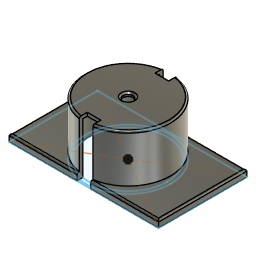
Magnet Holder v4 (Autodesk Fusion 360 design; units mm, degrees)
Autodesk Fusion 360 part; units mm, degrees
sketch "Sketch1" plane through (0, 0, 0) normal (0, 0, 1) x (1, 0, 0)
  circle A0 centre (0, 0) radius 11.5
  circle A1 centre (0, 0) radius 12.5
  line L0 (22, -13) -> (-22, -13)
  line L1 (-22, -13) -> (-22, 13)
  line L2 (-22, 13) -> (22, 13)
  line L3 (22, 13) -> (22, -13)
  line L4 (22, -13) -> (-22, 13) construction
  line L5 (-22, -13) -> (22, 13) construction
  constraint coincident A0.centre A1.centre
  constraint horizontal L0
  constraint perpendicular L0 L1
  constraint parallel L0 L2
  constraint parallel L1 L3
  constraint coincident L4 A0.centre
  constraint coincident L5 A0.centre
extrude "Extrude22" add sketch "Sketch1" along normal blind 2 contours A1 | L0 L1 L2 L3
sketch "Sketch16" plane through (0, 0, 2) normal (0, 0, 1) x (-1, 0, 0)
  circle A0 centre (0, 0) radius 11.5
  line L0 (-22, -13) -> (22, -13)
  line L1 (22, -13) -> (22, 13)
  line L2 (22, 13) -> (-22, 13)
  line L3 (-22, 13) -> (-22, -13)
  circle A1 centre (0, 0) radius 12.5
  constraint coincident A0.centre A1.centre
extrude "Extrude23" add sketch "Sketch16" along normal blind 13 contours A1
sketch "Sketch17" plane through (0, 0, 15) normal (0, 0, 1) x (-1, 0, 0)
  circle A0 centre (0, 0) radius 11.5
  circle A1 centre (0, 0) radius 12.5
  circle A2 centre (0, 0) radius 12.5
  constraint coincident A0.centre A1.centre
extrude "Extrude24" add sketch "Sketch17" along normal blind 1 contours A0 | A1 A2
hole "Hole3" at (0, 0, 16) direction (0, 0, -1) diameter 3 depth 6 tip angle 180 countersink diameter 4 countersink angle 90
sketch "Sketch18" plane through (0, 0, 16) normal (0, 0, 1) x (-1, 0, 0)
  circle A0 centre (0, 0) radius 2
  circle A1 centre (0, 0) radius 12.5
  line L0 (2, 10) -> (-2, 10)
  line L1 (-2, 10) -> (-2, 14)
  line L2 (-2, 14) -> (2, 14)
  line L3 (2, 14) -> (2, 10)
  line L4 (2, -10) -> (-2, -10)
  line L5 (-2, -10) -> (-2, -14)
  line L6 (-2, -14) -> (2, -14)
  line L7 (2, -14) -> (2, -10)
  constraint horizontal L0
  constraint vertical L1
  constraint horizontal L2
  constraint vertical L3
  constraint horizontal L4
  constraint vertical L5
  constraint horizontal L6
  constraint vertical L7
extrude "Extrude25" cut sketch "Sketch18" against normal blind 16 contours A1 L0 L1 L3 | A1 L1 L2 L3 | A1 L5 L6 L7 | A1 L4 L5 L7
fillet "Fillet3" radius 0.5 2 edges at (12.5, 0, 16) (-12.5, 0, 16)
fillet "Fillet4" radius 0.5 3 edges at (12, 13, 2) (22, 0, 2) (12, -13, 2)
fillet "Fillet5" radius 0.5 3 edges at (-12, -13, 2) (-22, 0, 2) (-12, 13, 2)
extrude "Extrude17" [rolled back] along distance 2 taper angle 0
extrude "Extrude18" [rolled back] along distance 15.24 taper angle 0
sketch "Sketch14" plane through (0, 0, 15.24) normal (0, 0, 1) x (-1, 0, 0)
  circle A0 centre (0, 0) radius 10
  circle A1 centre (0, 0) radius 11
  circle A2 centre (0, 0) radius 11
  constraint coincident A0.centre A1.centre
extrude "Extrude19" [rolled back] along distance 1 taper angle 0
hole "Hole2" [rolled back] hole depth 6 hole diameter 0.9 tip angle 180 csdiameter 2.5 csangle 90
sketch "Sketch15" plane through (0, 0, 16.24) normal (0, 0, 1) x (-1, 0, 0)
  circle A0 centre (0, 0) radius 1.25
  circle A1 centre (0, 0) radius 11
  line L0 (2, 9) -> (-2, 9)
  line L1 (-2, 9) -> (-2, 13)
  line L2 (-2, 13) -> (2, 13)
  line L3 (2, 13) -> (2, 9)
  line L4 (2, -9) -> (-2, -9)
  line L5 (-2, -9) -> (-2, -13)
  line L6 (-2, -13) -> (2, -13)
  line L7 (2, -13) -> (2, -9)
  constraint horizontal L0
  constraint vertical L1
  constraint horizontal L2
  constraint vertical L3
  constraint horizontal L4
  constraint vertical L5
  constraint horizontal L6
  constraint vertical L7
extrude "Extrude20" [rolled back] along distance -8 taper angle 0
fillet "Fillet1" [rolled back] radius 0.5
fillet "Fillet2" [rolled back] radius 0.5
extrude "Extrude21" [rolled back] along distance 2 taper angle 0
extrude "Extrude1" [rolled back] side1wall thickness 1 along distance 20 taper angle 0
sketch "Sketch2" plane through (0, 0, 0) normal (0, 0, 1) x (1, 0, 0)
  line L0 (-5, -10) -> (5, -10)
  line L1 (-5, -10) -> (-5, -8.6603)
  line L2 (5, -10) -> (5, -8.6603)
  arc A0 (5, -8.6603) -> (-5, -8.6603) centre (0, 0) ccw
  constraint horizontal L0
  constraint coincident A0.centre origin
  constraint perpendicular L0 L1
  constraint perpendicular L0 L2
extrude "Extrude2" [rolled back] along distance 2.5 taper angle 0
ref_plane "WorkPlane1" through (0, 0, 17.5) normal (0, 0, 1) x (1, 0, 0)
sketch "Sketch3" plane through (0, 0, 17.5) normal (0, 0, 1) x (1, 0, 0)
sketch "Sketch4" plane through (0, 0, 2.5) normal (0, 0, 1) x (-1, 0, 0)
  line L0 (5, 10) -> (-5, 10)
  line L1 (-5, 10) -> (-5, 8.6603)
  arc A0 (-5, 8.6603) -> (5, 8.6603) centre (0, 0) ccw
  line L2 (5, 8.6603) -> (5, 10)
  line L3 (-14, 9) -> (-6.3275, 9)
  line L4 (-14, 9) -> (-14, 5.5247)
  spline S0 degree 5 poles (-14, 5.5247) (-13.9496, 5.4874) (-13.8498, 5.4119) (-13.7027, 5.2958) (-13.512, 5.1353) (-13.283, 4.9251) (-13.0636, 4.7056) (-12.8545, 4.4775) (-12.6567, 4.242) (-12.4712, 4.0012) (-12.2993, 3.7572) (-12.1415, 3.5119) (-11.9978, 3.2656) (-11.8668, 3.0169) (-11.7458, 2.762) (-11.6318, 2.4964) (-11.5225, 2.2153) (-11.4171, 1.9151) (-11.3178, 1.5946) (-11.2257, 1.2533) (-11.1416, 0.8912) (-11.0809, 0.5849) (-11.039, 0.346) (-11.0127, 0.1827) (-11, 0.1) knots 0 0 0 0 0 0 0.05 0.1 0.15 0.2 0.25 0.3 0.35 0.4 0.45 0.5 0.55 0.6 0.65 0.7 0.75 0.8 0.85 0.9 0.95 1 1 1 1 1 1
  line L5 (-11.6858, 2.681) -> (-11.25, 1.43)
  spline S1 degree 5 poles (-6.3275, 9) (-6.5288, 8.8498) (-6.9165, 8.549) (-7.4534, 8.096) (-8.0838, 7.4871) (-8.7489, 6.709) (-9.3131, 5.9024) (-9.7954, 5.0559) (-10.2069, 4.1611) (-10.5469, 3.2164) (-10.8062, 2.224) (-10.9382, 1.3948) (-10.9888, 0.7544) (-11, 0.3195) (-11, 0.1) knots 0 0 0 0 0 0 0.1 0.2 0.3 0.4 0.5 0.6 0.7 0.8 0.9 1 1 1 1 1 1
  line L6 (-5.255, 9.8) -> (-7.4, 8.2)
  line L7 (-11, 1.3) -> (-11, -1.1)
  point P0 (-12.87, 4.49)
  point P1 (-12.0347, 3.325)
  point P2 (-11.4679, 2.0555)
  point P3 (-9.8, 5)
  constraint horizontal L3
  constraint perpendicular L3 L4
  constraint midpoint P2 L5
  constraint midpoint L3.end L6
  constraint midpoint S0.end L7
extrude "Extrude3" [rolled back] along distance 2 taper angle 0
sketch "Sketch5" plane through (0, 0, 2.5) normal (0, 0, 1) x (-1, 0, 0)
  line L0 (5, 10) -> (-5, 10)
  line L1 (-5, 10) -> (-5, 8.6603)
  arc A0 (-5, 8.6603) -> (5, 8.6603) centre (0, 0) ccw
  line L2 (5, 8.6603) -> (5, 10)
  line L3 (14, 9) -> (6.3249, 9)
  line L4 (14, 9) -> (14, 5.52)
  spline S0 degree 5 poles (10.9999, 0.073) (11.0319, 0.2346) (11.0981, 0.5527) (11.204, 1.0147) (11.3588, 1.5997) (11.5765, 2.2762) (11.8213, 2.8939) (12.0963, 3.4498) (12.4047, 3.9441) (12.748, 4.3849) (13.1266, 4.7859) (13.458, 5.0862) (13.7227, 5.305) (13.9064, 5.4487) (14, 5.52) knots 0 0 0 0 0 0 0.1 0.2 0.3 0.4 0.5 0.6 0.7 0.8 0.9 1 1 1 1 1 1
  line L5 (13.4267, 5.0834) -> (14.5733, 5.9566)
  spline S1 degree 5 poles (10.9999, 0.073) (11.0009, 0.2091) (10.9984, 0.4805) (10.9814, 0.8857) (10.9323, 1.4218) (10.826, 2.0845) (10.6756, 2.7386) (10.4831, 3.3819) (10.2565, 4.0106) (9.9997, 4.6218) (9.7097, 5.2156) (9.3805, 5.7931) (9.0049, 6.356) (8.5777, 6.9061) (8.097, 7.445) (7.5628, 7.9736) (7.0933, 8.3887) (6.7181, 8.696) (6.4577, 8.899) (6.3249, 9) knots 0 0 0 0 0 0 0.066667 0.133333 0.2 0.266667 0.333333 0.4 0.466667 0.533333 0.6 0.666667 0.733333 0.8 0.866667 0.933333 1 1 1 1 1 1
  line L6 (10.848, 2.2166) -> (10.152, 4.3834)
  point P0 (12.2, 3.6)
  point P1 (10.5, 3.3)
  point P2 (9.1, 6.2)
  constraint parallel L0 L3
  constraint perpendicular L3 L4
  constraint midpoint L4.end L5
  constraint midpoint P1 L6
extrude "Extrude4" [rolled back] along distance 2 taper angle 0
ref_plane "WorkPlane2" through (0, 0, 17.5) normal (0, 0, 1) x (1, 0, 0)
sketch "Sketch6" plane through (0, 0, 17.5) normal (0, 0, 1) x (1, 0, 0)
sketch "Sketch7" plane through (0, 0, 0) normal (0, 0, 1) x (1, 0, 0)
hole "Hole1" [rolled back] hole depth 2 hole diameter 3 tip angle 118 cbdepth 1 cbdiameter 4
extrude "Extrude5" [rolled back] along distance 2.5 taper angle 0
extrude "Extrude6" [rolled back] along distance 2.5 taper angle 0
extrude "Extrude7" [rolled back] along distance -2 taper angle 0
extrude "Extrude8" [rolled back] along distance -2 taper angle 0
ref_plane "WorkPlane3" through (0, 0, 17.5) normal (0, 0, 1) x (1, 0, 0)
sketch "Sketch8" plane through (0, 0, 17.5) normal (0, 0, 1) x (1, 0, 0)
  line L0 (-14, -9) -> (-6.3251, -9)
  line L1 (-14, -9) -> (-14, -5.5188)
  spline S0 degree 5 poles (-14, -5.5188) (-13.9096, -5.4464) (-13.7383, -5.3073) (-13.5098, -5.1161) (-13.2493, -4.8848) (-12.9385, -4.5749) (-12.5913, -4.1764) (-12.1926, -3.6334) (-11.8154, -2.9315) (-11.4931, -2.1293) (-11.2439, -1.3171) (-11.1073, -0.7399) (-11.0401, -0.3851) (-11.0108, -0.1884) (-11, -0.1) knots 0 0 0 0 0 0 0.1 0.2 0.3 0.4 0.5 0.6 0.7 0.8 0.9 1 1 1 1 1 1
  line L2 (-14.61, -6.0076) -> (-13.39, -5.03)
  line L3 (-12.8121, -4.4826) -> (-11.9879, -3.3174)
  line L4 (-11.05, -0.51) -> (-10.95, 0.31)
  spline S1 degree 5 poles (-11, -0.1) (-10.9944, -0.2588) (-10.9791, -0.5743) (-10.9436, -1.0413) (-10.871, -1.6515) (-10.7372, -2.3925) (-10.5591, -3.1106) (-10.3363, -3.8043) (-10.0691, -4.4715) (-9.7604, -5.1102) (-9.4143, -5.7181) (-9.0362, -6.2933) (-8.6311, -6.8339) (-8.2039, -7.3388) (-7.758, -7.8078) (-7.296, -8.2418) (-6.9147, -8.5617) (-6.6223, -8.7866) (-6.4246, -8.93) (-6.3251, -9) knots 0 0 0 0 0 0 0.066667 0.133333 0.2 0.266667 0.333333 0.4 0.466667 0.533333 0.6 0.666667 0.733333 0.8 0.866667 0.933333 1 1 1 1 1 1
  point P0 (-12.4, -3.9)
  point P1 (-10.25, -4)
  point P2 (-8.5, -6.98)
  constraint horizontal L0
  constraint perpendicular L0 L1
  constraint midpoint L1.end L2
  constraint midpoint P0 L3
  constraint midpoint S0.end L4
extrude "Extrude9" [rolled back] along distance 2.5 taper angle 0
ref_plane "WorkPlane4" through (0, 0, 17.5) normal (0, 0, 1) x (1, 0, 0)
sketch "Sketch9" plane through (0, 0, 17.5) normal (0, 0, 1) x (1, 0, 0)
ref_plane "WorkPlane5" through (0, 0, 17.5) normal (0, 0, 1) x (1, 0, 0)
sketch "Sketch10" plane through (0, 0, 17.5) normal (0, 0, 1) x (1, 0, 0)
extrude "Extrude10" [rolled back] along distance 2.5 taper angle 0
extrude "Extrude11" [rolled back] along distance 2.5 taper angle 0
extrude "Extrude12" [rolled back] along distance 2.5 taper angle 0
sketch "Sketch11" plane through (0, 0, 10) normal (0, 0, 1) x (-1, 0, 0)
  arc A0 (-6.3778, 8.9623) -> (-8.6399, 6.8082) centre (0, 0) ccw
  spline S0 degree 5 poles (-6.3778, 8.9623) (-6.3678, 8.9699) (-6.3578, 8.9774) (-6.3477, 8.9849) (-6.3376, 8.9925) (-6.3275, 9) knots -0.005017 -0.005017 -0.005017 -0.005017 -0.005017 -0.005017 0 0 0 0 0 0
  line L0 (-6.3275, 9) -> (-14, 9)
  line L1 (-14, 9) -> (-14, 5.5247)
  spline S1 degree 5 poles (-14, 5.5247) (-13.9496, 5.4874) (-13.8498, 5.4119) (-13.7027, 5.2958) (-13.5138, 5.1367) (-13.3321, 4.9701) (-13.2005, 4.8415) (-13.1153, 4.7546) (-13.0739, 4.7115) knots 0 0 0 0 0 0 0.05 0.1 0.15 0.198199 0.198199 0.198199 0.198199 0.198199 0.198199
  spline S2 degree 3 poles (-11.2557, 1.3573) (-11.4192, 1.9852) (-11.676, 2.7302) (-12.3168, 3.8089) (-12.6229, 4.2482) (-13.0739, 4.7115) knots -0.846571 -0.846571 -0.846571 -0.846571 -0.372929 -0.372929 -0.135747 -0.135747 -0.135747 -0.135747
  spline S3 degree 5 poles (-11.2557, 1.3573) (-11.25, 1.3356) (-11.2264, 1.2445) (-11.186, 1.0809) (-11.1312, 0.8386) (-11.0809, 0.5849) (-11.039, 0.346) (-11.0127, 0.1827) (-11, 0.1) knots 0.834334 0.834334 0.834334 0.834334 0.834334 0.834334 0.85 0.9 0.95 1 1 1 1 1 1
  spline S4 degree 5 poles (-11, 0.1) (-11, 0.3195) (-10.9888, 0.7544) (-10.9382, 1.3948) (-10.8062, 2.224) (-10.5469, 3.2164) (-10.2069, 4.1611) (-9.7954, 5.0559) (-9.3966, 5.7558) (-9.0541, 6.2669) (-8.799, 6.6076) (-8.6569, 6.787) (-8.6399, 6.8082) knots -1 -1 -1 -1 -1 -1 -0.9 -0.8 -0.7 -0.6 -0.5 -0.4 -0.3 -0.286569 -0.286569 -0.286569 -0.286569 -0.286569 -0.286569
extrude "Extrude13" [rolled back] along distance 2.5 taper angle 0
extrude "Extrude14" [rolled back] along distance 5 taper angle 0
extrude "Extrude15" [rolled back] along distance 2.5 taper angle 0
sketch "Sketch12" plane through (0, 0, 0) normal (1, 0, 0) x (0, 1, 0)
sketch "Sketch13" plane through (0, 0, 0) normal (1, 0, 0) x (0, 1, 0)
  circle A0 centre (3.5, 5.5) radius 1.75
extrude "Extrude16" [rolled back] along distance 20 taper angle 0 against distance 16 side2taper angle 0
